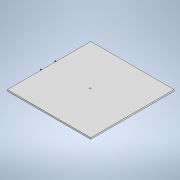
# Autodesk Inventor part: cube lid
Saved by Autodesk Inventor 2021 (Build 250183000, 183)
## iProperties
Created: 2021-07-23
Part Number: cube lid
Material: Generic
Document SubType Name: Modeling
Designer: Nishat
Density: 1 g/cm^3
Appearance: Default
Author: Nishat
Autodesk Inventor part; units mm, degrees
ref_plane "YZ Plane" through (0, 0, 0) normal (1, 0, 0) x (0, 1, 0)
ref_plane "XZ Plane" through (0, 0, 0) normal (0, 1, 0) x (-1, 0, 0)
ref_plane "XY Plane" through (0, 0, 0) normal (0, 0, 1) x (1, 0, 0)
sketch "Sketch1" plane through (0, 0, 0) normal (0, 1, 0) x (-1, 0, 0)
  line L0 (1400, 1400) -> (-1400, 1400)
  line L1 (-1400, 1400) -> (-1400, -1400)
  line L2 (-1400, -1400) -> (1400, -1400)
  line L3 (1400, -1400) -> (1400, 1400)
  point P0 (0, 0)
  dimension "d0" = 2800
  dimension "d1" = 2800
  dimension "d2" = 1400
  dimension "d3" = 1400
  constraints: 8 end point, 2 parallel, 1 horizontal, 1 perpendicular
  measures "d0" distance of L2.end L0.start
  measures "d1" distance between parallel lines of L1 L3
  measures "d2" distance from line of L1 point (0, 0)
  measures "d3" distance from line of L0 point (0, 0)
extrude "Extrusion1" add sketch "Sketch1" along normal blind 50
sketch "Sketch2" plane through (-1400, 0, -1400) normal (-1, 0, 0) x (0, 0, 1)
  line L0 (2800, 50) -> (0, 50) projected
  line L1 (2800, 0) -> (0, 0) projected
  line L2 (1150, 50) -> (1650, 50)
  line L3 (1650, 50) -> (1650, 0)
  line L4 (1650, 0) -> (1150, 0)
  line L5 (1150, 0) -> (1150, 50)
  line L6 (0, 0) -> (0, 50) projected
  point P0 (1400, 0)
  dimension "d6" = 500
  dimension "d7" = 1150
  constraints: 8 end point, 2 parallel, 2 point on line, 1 horizontal, 1 perpendicular
  measures "d6" distance between parallel lines of L3 L5
  measures "d7" distance between parallel lines of L5 L6
extrude "Extrusion2" add sketch "Sketch2" along normal blind 50 contours L3 L1 L5 L0
sketch "Sketch4" plane through (-1450, 0, -1400) normal (-1, 0, 0) x (0, 0, 1)
  line L0 (2800, 0) -> (0, 0) projected
  line L1 (1160, 50) -> (1640, 50)
  line L2 (1640, 50) -> (1640, 0)
  line L3 (1640, 0) -> (1160, 0)
  line L4 (1160, 0) -> (1160, 50)
  line L5 (1650, 50) -> (1150, 50) projected
  line L6 (1150, 50) -> (1150, 0) projected
  line L7 (1650, 0) -> (1650, 50) projected
  point P0 (1400, 0)
  point P1 (1160, 0)
  dimension "d10" = 0
  dimension "d11" = 10
  dimension "d12" = 10
  constraints: 8 end point, 2 parallel, 1 horizontal, 1 perpendicular, 1 point on line
  measures "d10" distance between parallel lines of L5 L1
  measures "d11" distance between parallel lines of L4 L6
  measures "d12" distance between parallel lines of L7 L2
extrude "Extrusion3" cut sketch "Sketch4" against normal blind 50 contours L0 L4 L1 L2
sketch "Sketch5" plane through (-1400, 0, 250) normal (0, 0, 1) x (1, 0, 0)
  circle A0 centre (-25, 26.8195) radius 15
  line L0 (-50, 0) -> (-50, 50) projected
  point P0 (1400, 0)
  dimension "d15" = 30
  dimension "d16" = 25
  constraints: 1 centre point
  measures "d15" diameter of A0
  measures "d16" distance from line of A0.centre L0
extrude "Extrusion4" cut sketch "Sketch5" against normal blind 700
sketch "Sketch6" plane through (-1400, 0, -1400) normal (-1, 0, 0) x (0, 0, 1)
  point P0 (1400, 0)
body "Solid1"
